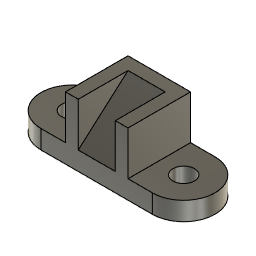
A2 v1 (Autodesk Fusion 360 design; units mm, degrees)
Autodesk Fusion 360 part; units mm, degrees
sketch "base" plane through (0, 0, 0) normal (0, 0, 1) x (1, 0, 0)
  line L0 (-35, -17) -> (79, -17)
  line L1 (79, 47) -> (-35, 47)
  circle A0 centre (-35, 15) radius 11
  circle A1 centre (79, 15) radius 11
  arc A2 (79, -17) -> (79, 47) centre (79, 15) ccw
  arc A3 (-35, 47) -> (-35, -17) centre (-35, 15) ccw
  dimension "d1" = 114
  dimension "d2" = 64
  dimension "d3" = 22
  dimension "d4" = 22
  constraint horizontal L0
  constraint horizontal L1
  constraint tangent L1 A2
  constraint tangent L1 A3
  measures "d1" distance of L0.start L0.end
  measures "d2" distance of L0.start L1.end
  measures "d3" diameter of A0
  measures "d4" diameter of A1
extrude "Extrude1" add sketch "base" along normal blind 19
sketch "middle" plane through (0, 0, 19) normal (0, 0, 1) x (-1, 0, 0)
  circle A0 centre (-79, -15) radius 11
  circle A1 centre (35, -15) radius 11
  arc A2 (35, -47) -> (35, 17) centre (35, -15) ccw
  line L0 (35, 17) -> (-79, 17)
  arc A3 (-79, 17) -> (-79, -47) centre (-79, -15) ccw
  line L1 (-79, -47) -> (35, -47)
  line L2 (-22, -47) -> (-3, -47)
  line L3 (-22, -47) -> (-41, -47)
  line L4 (-22, -47) -> (-54, -47)
  line L5 (-22, -47) -> (10, -47)
  line L6 (10, -47) -> (10, 17)
  line L7 (10, 17) -> (-3.0614, 17)
  line L8 (-3.0614, 17) -> (-3.0614, -34)
  line L9 (-54, -47) -> (-54, 17)
  line L10 (-54, 17) -> (-41, 17)
  line L11 (-41, 17) -> (-41, -34)
  line L12 (-41, -34) -> (-3.0614, -34)
  dimension "d10" = 32
  dimension "d11" = 32
  dimension "d12" = 51
  constraint midpoint L1 L2.start
  constraint coincident L1 L2.end
  constraint parallel L1 L2
  constraint coincident L1 L3.end
  constraint parallel L1 L4
  constraint parallel L1 L5
  constraint coincident L0 L6.end
  constraint perpendicular L0 L6
  constraint coincident L0 L7.end
  constraint perpendicular L7 L8
  constraint coincident L0 L9.end
  constraint perpendicular L0 L9
  constraint coincident L0 L10.end
  constraint perpendicular L10 L11
  constraint perpendicular L8 L12
  measures "d10" distance of L2.start L4.end
  measures "d11" distance of L2.start L5.end
  measures "d12" distance of L7.end L8.end
extrude "Extrude2" add sketch "middle" along normal blind 45 contours L0 L8 L11 L12
sketch "ramp" plane through (41, 0, 0) normal (1, 0, 0) x (0, 1, 0)
  line L0 (-17, 19) -> (34, 19)
  line L1 (34, 19) -> (34, 64)
  line L2 (34, 64) -> (-17, 64)
  line L3 (-17, 64) -> (-17, 19)
  line L4 (34, 64) -> (-17, 19)
  line L5 (-17, 64) -> (-17, 19)
  line L6 (-17, 64) -> (34, 64)
  constraint coincident L1.end L2.start
  constraint coincident L0.start L3.end
  constraint coincident L2.end L3.start
extrude "Extrude3" cut sketch "ramp" against normal blind 38 contours L2 L3 L4 L5 L6
extrude "Extrude4" add sketch "middle" along normal blind 45 contours L0 L1 L2 L3 L4 L5 L6 L7 L8 L9 L10 L11 L12
